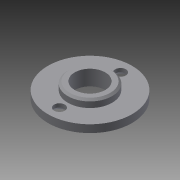
# Autodesk Inventor part: Крышка
Saved by Autodesk Inventor 2015 SP1 (Build 190203100, 203)
## iProperties
Created: 2019-05-12
Part Number: Крышка
Material: Типовые
Document SubType Name: Modeling
Density: 1 g/cm^3
Appearance: По умолчанию
Autodesk Inventor part; units mm, degrees
ref_plane "YZ Plane" through (0, 0, 0) normal (1, 0, 0) x (0, 1, 0)
ref_plane "XZ Plane" through (0, 0, 0) normal (0, 1, 0) x (-1, 0, 0)
ref_plane "XY Plane" through (0, 0, 0) normal (0, 0, 1) x (1, 0, 0)
sketch "Эскиз1" plane through (0, 0, 0) normal (0, 0, 1) x (1, 0, 0)
  circle A0 centre (0, 0) radius 55
  circle A1 centre (0, 0) radius 20
  circle A2 centre (0, 40) radius 7
  circle A3 centre (0, -40) radius 7
  dimension "d0" = 110
  dimension "d1" = 40
  dimension "d3" = 14
  dimension "d6" = 360
  constraints: 4 centre point, 4 coincident, 5 other
  measures "d0" diameter of A0
  measures "d1" diameter of A1
  measures "d3" diameter of A2
extrude "Выдавливание1" add sketch "Эскиз1" along normal blind 20
sketch "Эскиз2" plane through (0, 0, 20) normal (0, 0, 1) x (1, 0, 0)
  circle A0 centre (0, 0) radius 55 projected
  circle A1 centre (0, 0) radius 29
  dimension "d10" = 58
  constraints: 1 centre point, 1 coincident
  measures "d10" diameter of A1
extrude "Выдавливание2" cut sketch "Эскиз2" against normal blind 10
chamfer "Фаска1" distance 2.5 angle 45 1 edges at (-29, 0, 20)
chamfer "Фаска2" distance 5.2 angle 45 1 edges at (-7, -40, 0)
chamfer "Фаска3" distance 5.2 angle 45 1 edges at (-7, 40, 0)
